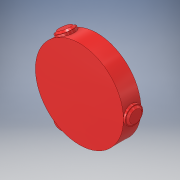
# Autodesk Inventor part: Platform
Saved by Autodesk Inventor 2019 (Build 230136000, 136)
## iProperties
Created: 2022-07-06
Part Number: Platform
Material: Generic
Document SubType Name: Modeling
Designer: zreik
Density: 1 g/cm^3
Appearance: Light Red
Author: zreik
Autodesk Inventor part; units mm, degrees
ref_plane "XZ Plane" through (0, 0, 0) normal (0, 1, 0) x (-1, 0, 0)
ref_plane "XY Plane" through (0, 0, 0) normal (0, 0, 1) x (1, 0, 0)
sketch "Sketch1" plane through (0, 0, 0) normal (0, 0, 1) x (1, 0, 0)
  circle A0 centre (0, 0) radius 25
  dimension "d0" = 50
  constraints: 1 centre point, 1 coincident
  measures "d0" diameter of A0
extrude "Extrusion1" add sketch "Sketch1" along normal mid plane 10
ref_plane "Work Plane1" through (25, 0, 0) normal (1, 0, 0) x (0, 1, 0)
sketch "Sketch2" plane through (25, 0, 0) normal (1, 0, 0) x (0, 1, 0)
  circle A0 centre (0, 0) radius 5
  line L0 (-25, -5) -> (25, -5) projected
  point P0 (0, 0)
  constraints: 1 centre point, 1 coincident, 1 tangent
extrude "Extrusion2" add sketch "Sketch2" along normal mid plane 2
sketch "Sketch3" plane through (26, 0, 0) normal (1, 0, 0) x (0, 0, -1)
  circle A0 centre (0, 0) radius 3.5
  point P0 (0, 0)
  dimension "d5" = 7
  constraints: 1 centre point, 1 coincident
  measures "d5" diameter of A0
extrude "Extrusion3" add sketch "Sketch3" along normal blind 1
chamfer "Chamfer1" distance 1 angle 45 1 edges at (26, 0, 3.5)
pattern_circular "Circular Pattern1" count 3 over 360 about axis through (0, 0, 0) along (0, 0, 1) of "Extrusion2", "Extrusion3", "Chamfer1"
body "Solid1"
